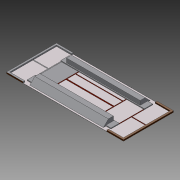
# Autodesk Inventor part: Ball Field
Saved by Autodesk Inventor 2015 (Build 190159000, 159)
## iProperties
Created: 2016-11-29
Part Number: Ball Field
Material: Generic
Document SubType Name: Modeling
Designer: Simms
Density: 1 g/cm^3
Appearance: Default
Author: Simms
Autodesk Inventor part; units mm, degrees
ref_plane "YZ Plane" through (0, 0, 0) normal (1, 0, 0) x (0, 1, 0)
ref_plane "XZ Plane" through (0, 0, 0) normal (0, 1, 0) x (-1, 0, 0)
ref_plane "XY Plane" through (0, 0, 0) normal (0, 0, 1) x (1, 0, 0)
sketch "Sketch1" plane through (0, 0, 0) normal (0, 1, 0) x (-1, 0, 0)
  line L0 (0, 381) -> (-889, 381)
  line L1 (-889, 381) -> (-889, -381)
  line L2 (-889, -381) -> (0, -381)
  line L3 (0, 381) -> (0, -381)
  point P0 (0, 0)
  dimension "d1" = 762
  dimension "d35" = 889
  constraints: 8 end point, 1 horizontal, 1 parallel, 1 perpendicular
  measures "d1" distance of L1.end L0.end
  measures "d35" distance between parallel lines of L1 L3
extrude "Extrusion1" add sketch "Sketch1" along normal blind 2.54
sketch "Sketch2" plane through (0, 2.54, 0) normal (0, 1, 0) x (1, 0, 0)
  line L0 (0, -381) -> (889, -381) projected
  line L1 (889, -381) -> (889, 381) projected
  line L2 (889, 381) -> (0, 381) projected
  line L3 (863.6, -355.6) -> (635, -355.6)
  line L4 (635, 355.6) -> (863.6, 355.6)
  line L5 (863.6, 355.6) -> (863.6, -355.6)
  line L6 (635, -381) -> (635, -355.6)
  line L7 (635, 355.6) -> (635, 381)
  line L8 (0, 381) -> (0, -381) projected
  line L9 (635, -355.6) -> (635, 355.6) construction
  line L10 (622.3, 190.5) -> (622.3, -190.5)
  line L11 (863.6, 6.35) -> (863.6, -6.35)
  line L12 (863.6, -6.35) -> (635, -6.35)
  line L13 (635, -190.5) -> (635, -6.35)
  line L14 (635, 6.35) -> (635, 190.5)
  line L15 (635, 6.35) -> (863.6, 6.35)
  line L16 (0, -190.5) -> (0, -317.5)
  line L17 (0, -317.5) -> (635, -317.5)
  line L18 (635, -317.5) -> (635, -190.5)
  line L19 (622.3, -190.5) -> (0, -190.5)
  line L20 (0, 0) -> (889, 0) construction
  line L21 (0, 190.5) -> (0, 317.5)
  line L22 (0, 317.5) -> (635, 317.5)
  line L23 (635, 317.5) -> (635, 190.5)
  line L24 (622.3, 190.5) -> (0, 190.5)
  line L25 (368.3, 190.5) -> (368.3, -190.5)
  line L26 (622.3, -190.5) -> (635, -190.5)
  line L27 (622.3, 190.5) -> (635, 190.5)
  line L28 (0, 0) -> (1199.5673, 0) construction
  line L29 (355.6, -9.525) -> (0, -9.525)
  line L30 (0, -9.525) -> (0, 9.525)
  line L31 (0, 9.525) -> (355.6, 9.525)
  line L32 (0, 133.35) -> (355.6, 133.35)
  line L33 (0, 146.05) -> (0, 133.35)
  line L34 (355.6, 146.05) -> (0, 146.05)
  line L35 (355.6, 9.525) -> (355.6, 133.35)
  line L36 (355.6, 146.05) -> (355.6, 190.5)
  line L37 (0, -133.35) -> (355.6, -133.35)
  line L38 (0, -146.05) -> (0, -133.35)
  line L39 (355.6, -146.05) -> (0, -146.05)
  line L40 (355.6, -190.5) -> (355.6, -146.05)
  line L41 (355.6, -133.35) -> (355.6, -9.525)
  line L42 (635, -381) -> (889, -381)
  line L43 (889, -381) -> (889, 381)
  line L44 (889, 381) -> (635, 381)
  line L45 (889, 381) -> (0, 381) projected
  point P0 (745.8337, 0)
  point P1 (599.7837, 0)
  point P2 (345.7837, 88.9)
  dimension "d4" = 25.4
  dimension "d5" = 254
  dimension "d8" = 12.7
  dimension "d11" = 127
  dimension "d16" = 19.05
  dimension "d19" = 63.5
  dimension "d21" = 44.45
  dimension "d22" = 12.7
  dimension "d23" = 374.65
  dimension "d36" = 25.4
  dimension "d37" = 0
  dimension "d38" = 0
  dimension "d39" = 0
  dimension "d40" = 0
  dimension "d41" = 254
  dimension "d42" = 12.7
  dimension "d43" = 12.7
  dimension "d44" = 0
  dimension "d45" = 12.7
  dimension "d46" = 0
  dimension "d47" = 12.7
  constraints: 83 end point, 11 parallel, 6 horizontal, 4 point on line, 3 collinear, 3 perpendicular, 2 midpoint, 1 vertical
  measures "d4" distance between parallel lines of L0 L3
  measures "d5" distance from line of L3.end L1
  measures "d8" distance of L10.start L14.end
  measures "d11" distance of L16.end L16.start
  measures "d16" distance of L29.end L30.end
  measures "d19" distance between parallel lines of L17 L0
  measures "d21" distance between parallel lines of L24 L34
  measures "d22" distance between parallel lines of L15 L12
  measures "d23" distance between parallel lines of L12 L0
  measures "d36" distance between parallel lines of L5 L1
  measures "d37" distance between parallel lines of L5 L11
  measures "d38" distance between parallel lines of L18 L9
  measures "d39" distance between parallel lines of L9 L14
  measures "d40" distance between parallel lines of L8 L16
  measures "d41" distance between parallel lines of L10 L25
  measures "d42" distance between parallel lines of L25 L40
  measures "d43" distance between parallel lines of L25 L36
  measures "d44" distance between parallel lines of L8 L30
  measures "d45" distance between parallel lines of L25 L35
  measures "d46" distance between parallel lines of L8 L38
  measures "d47" distance between parallel lines of L25 L41
extrude "Extrusion2" add sketch "Sketch2" along normal blind 12.7 contours L8 L19 L26 L18 L17 | L24 L8 L22 L23 L27
extrude "Extrusion3" add sketch "Sketch2" along normal blind 19.05 contours L6 L3 L5 L4 L7 L2 L1 L0
extrude "Extrusion4" add sketch "Sketch2" along normal blind 0.254 contours L8 L37 L41 L29 L31 L35 L32 L34 L36 L24 L25 L19 L40 L39 | L26 L10 L27 L14 L15 L5 L12 L13
sketch "Sketch3" plane through (0, 0, -381) normal (-1, 0, 0) x (0, 0, 1)
  line L0 (762, 0) -> (0, 0) projected
  line L1 (762, 0) -> (762, 2.54) projected
  line L2 (698.5, 2.54) -> (762, 2.54) projected
  line L3 (698.5, 2.54) -> (698.5, 15.24) projected
  line L4 (571.5, 15.24) -> (698.5, 15.24) projected
  line L5 (571.5, 2.54) -> (571.5, 15.24) projected
  line L6 (527.05, 2.54) -> (571.5, 2.54) projected
  line L7 (527.05, 2.54) -> (527.05, 2.794) projected
  line L8 (514.35, 2.794) -> (527.05, 2.794) projected
  line L9 (514.35, 2.54) -> (514.35, 2.794) projected
  line L10 (390.525, 2.54) -> (514.35, 2.54) projected
  line L11 (390.525, 2.54) -> (390.525, 2.794) projected
  line L12 (371.475, 2.794) -> (390.525, 2.794) projected
  line L13 (371.475, 2.54) -> (371.475, 2.794) projected
  line L14 (247.65, 2.54) -> (371.475, 2.54) projected
  line L15 (247.65, 2.54) -> (247.65, 2.794) projected
  line L16 (234.95, 2.794) -> (247.65, 2.794) projected
  line L17 (234.95, 2.54) -> (234.95, 2.794) projected
  line L18 (190.5, 2.54) -> (234.95, 2.54) projected
  line L19 (190.5, 2.54) -> (190.5, 15.24) projected
  line L20 (63.5, 15.24) -> (190.5, 15.24) projected
  line L21 (63.5, 2.54) -> (63.5, 15.24) projected
  line L22 (0, 2.54) -> (63.5, 2.54) projected
  line L23 (0, 0) -> (0, 2.54) projected
  line L24 (736.6, 2.54) -> (584.2, 2.54)
  line L25 (387.35, 2.54) -> (698.5, 2.54) projected
  line L26 (736.6, 2.54) -> (889, 2.54) construction
  line L27 (736.6, 2.54) -> (660.4, 78.74)
  line L28 (736.6, 2.54) -> (844.3631, 2.54) construction
  line L29 (660.4, 78.74) -> (584.2, 78.74)
  line L30 (762, 0) -> (0, 0) projected
  line L31 (584.2, 78.74) -> (584.2, 2.54)
  line L32 (381, 2.54) -> (381, -13.3549) construction
  line L33 (25.4, 2.54) -> (177.8, 2.54)
  line L34 (374.65, 2.54) -> (63.5, 2.54)
  line L35 (25.4, 2.54) -> (101.6, 78.74)
  line L36 (101.6, 78.74) -> (177.8, 78.74)
  line L37 (177.8, 78.74) -> (177.8, 2.54)
  point P0 (381, 0)
  dimension "d30" = 152.4
  dimension "d31" = 180
  dimension "d32" = 135
  constraints: 24 end point, 5 symmetric about line, 2 equal length, 2 horizontal, 1 collinear, 1 parallel, 1 perpendicular, 1 vertical
  measures "d30" distance of L24.start L24.end
  measures "d31" angle of L24 L26
  measures "d32" angle of L28 L27
extrude "Extrusion5" add sketch "Sketch3" against normal blind 558.8 contours L2 L3 L4 L31 L29 L27 | L35 L36 L37 L20 L21 L22 | L24 L31 L4 L3 | L21 L20 L37 L33
mirror "Mirror1" about plane through (0, 0, 0) normal (1, 0, 0) of "Extrusion1", "Extrusion2", "Extrusion3", "Extrusion4", "Extrusion5"
body "Solid1"
